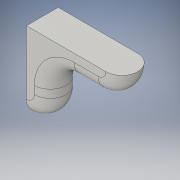
# Autodesk Inventor part: shelfBracket
Saved by Autodesk Inventor 2016 (Build 200138000, 138)
## iProperties
Created: 2015-09-21
Part Number: shelfBracket
Material: Generic
Document SubType Name: Modeling
Designer: xdlea
Density: 1 g/cm^3
Appearance: Smooth - White
Author: xdlea
Autodesk Inventor part; units mm, degrees
ref_plane "YZ Plane" through (0, 0, 0) normal (1, 0, 0) x (0, 1, 0)
ref_plane "XZ Plane" through (0, 0, 0) normal (0, 1, 0) x (-1, 0, 0)
ref_plane "XY Plane" through (0, 0, 0) normal (0, 0, 1) x (1, 0, 0)
sketch "Sketch1" plane through (0, 0, 0) normal (0, 0, 1) x (1, 0, 0)
  line L0 (0, 0) -> (114.3, 0)
  line L1 (114.3, 0) -> (114.3, 38.1)
  line L2 (114.3, 38.1) -> (-38.1, 38.1)
  line L3 (-38.1, 38.1) -> (-38.1, -88.9)
  line L4 (-38.1, -88.9) -> (0, -88.9)
  line L5 (0, -88.9) -> (0, 0)
  dimension "d0" = 152.4
  dimension "d1" = 127
  dimension "d2" = 38.1
  dimension "d3" = 38.1
  constraints: 12 end point, 5 perpendicular, 1 horizontal
  measures "d0" distance of L1.end L2.end
  measures "d1" distance of L2.end L3.end
  measures "d2" distance between parallel lines of L0 L2
  measures "d3" distance of L3.end L4.end
extrude "Extrusion1" add sketch "Sketch1" along normal mid plane 50.8
fillet "Fillet1" radius 38.1 3 edges at (0, -88.9, 0) (114.3, 0, 0) (0, 0, 0)
fillet "Fillet2" radius 25.4 8 edges at (0, -44.45, 25.4) (-11.1591, -77.7409, 25.4) (57.15, 0, 25.4) (103.1409, 11.1591, 25.4) (57.15, 0, -25.4) (103.1409, 11.1591, -25.4) (-11.1591, -77.7409, -25.4) (0, -44.45, -25.4)
body "Solid1"
